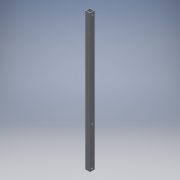
# Autodesk Inventor part: 1x1 8th Inch Aluminum Tube Custom Lift Arms
Saved by Autodesk Inventor 2016 (Build 200138000, 138)
## iProperties
Created: 2016-01-28
Part Number: 1x1 8th Inch Aluminum Tube Custom Lift Arms
Material: Generic
Document SubType Name: Modeling
Designer: Jack Jaworski
Density: 1 g/cm^3
Appearance: Default
Author: Jack Jaworski
Autodesk Inventor part; units mm, degrees
ref_plane "YZ Plane" through (0, 0, 0) normal (1, 0, 0) x (0, 1, 0)
ref_plane "XZ Plane" through (0, 0, 0) normal (0, 1, 0) x (-1, 0, 0)
ref_plane "XY Plane" through (0, 0, 0) normal (0, 0, 1) x (1, 0, 0)
sketch "Sketch1" plane through (0, 0, 0) normal (0, 1, 0) x (-1, 0, 0)
  line L0 (0, 0) -> (25.4, 0)
  line L1 (25.4, 0) -> (25.4, 25.4)
  line L2 (25.4, 25.4) -> (0, 25.4)
  line L3 (0, 25.4) -> (0, 0)
  line L4 (3.175, 3.175) -> (22.225, 3.175)
  line L5 (22.225, 3.175) -> (22.225, 22.225)
  line L6 (22.225, 22.225) -> (3.175, 22.225)
  line L7 (3.175, 22.225) -> (3.175, 3.175)
  dimension "d0" = 25.4
  dimension "d1" = 25.4
  dimension "d2" = 3.175
  dimension "d3" = 3.175
  dimension "d4" = 3.175
  dimension "d6" = 3.175
  constraints: 16 end point, 4 parallel, 2 horizontal, 2 perpendicular
  measures "d0" distance of L0.end L1.end
  measures "d1" distance of L1.end L2.end
  measures "d2" distance between parallel lines of L1 L5
  measures "d3" distance between parallel lines of L2 L6
  measures "d4" distance between parallel lines of L3 L7
  measures "d6" distance between parallel lines of L0 L4
extrude "Extrusion1" add sketch "Sketch1" along normal blind 762
sketch "Sketch3" plane through (0, 0, 25.4) normal (1, 0, 0) x (0, 0, -1)
  circle A0 centre (12.7, 12.7) radius 5.08
  line L0 (25.4, 0) -> (25.4, 762) projected
  line L1 (0, 0) -> (25.4, 0) projected
  dimension "d17" = 10.16
  dimension "d18" = 12.7
  dimension "d19" = 12.7
  constraints: 1 centre point
  measures "d17" diameter of A0
  measures "d18" distance from line of L0 A0.centre
  measures "d19" distance from line of L1 A0.centre
extrude "Extrusion3" cut sketch "Sketch3" against normal blind 25.4
sketch "Sketch4" plane through (0, 0, 25.4) normal (1, 0, 0) x (0, 0, -1)
  line L0 (0, 0) -> (0, 762) projected
  line L1 (0, 0) -> (25.4, 0) projected
  line L2 (25.4, 0) -> (25.4, 762) projected
  point P0 (12.7, 12.7)
  dimension "d22" = 12.7
  dimension "d23" = 12.7
  measures "d22" distance from line of L0 point (12.7, 12.7)
  measures "d23" distance from line of L1 point (12.7, 12.7)
sketch "Sketch5" plane through (0, 0, 25.4) normal (1, 0, 0) x (0, 0, -1)
  line L0 (15.4496, 744.5375) -> (9.9504, 744.5375)
  line L1 (9.9504, 744.5375) -> (7.2007, 749.3)
  line L2 (7.2007, 749.3) -> (9.9504, 754.0625)
  line L3 (9.9504, 754.0625) -> (15.4496, 754.0625)
  line L4 (15.4496, 754.0625) -> (18.1993, 749.3)
  line L5 (18.1993, 749.3) -> (15.4496, 744.5375)
  line L6 (0, 0) -> (0, 762) projected
  line L7 (0, 762) -> (25.4, 762) projected
  point P0 (25.4, 0)
  point P1 (12.7, 749.3)
  point P2 (12.7, 744.5375)
  dimension "d29" = 9.525
  dimension "d30" = 12.7
  dimension "d31" = 12.7
  constraints: 12 end point, 1 horizontal, 1 midpoint, 13 other
  measures "d29" distance between parallel lines of L0 L3
  measures "d30" distance from line of L6 point (12.7, 749.3)
  measures "d31" distance from line of L7 point (12.7, 749.3)
extrude "Extrusion5" cut sketch "Sketch5" against normal blind 25.4
extrude "Extrusion7" [suppressed]
sketch "Sketch6" plane through (0, 0, 25.4) normal (1, 0, 0) x (0, 0, -1)
  circle A0 centre (12.7, 226.06) radius 11.1125
  line L0 (25.4, 0) -> (25.4, 762) projected
  line L1 (0, 0) -> (25.4, 0) projected
  dimension "d40" = 22.225
  dimension "d41" = 12.7
  dimension "d42" = 226.06
  constraints: 1 centre point
  measures "d40" diameter of A0
  measures "d41" distance from line of L0 A0.centre
  measures "d42" distance from line of A0.centre L1
extrude "Extrusion8" cut sketch "Sketch6" against normal blind 25.4
equation "\"d4\" = d2"
body "Solid1"
